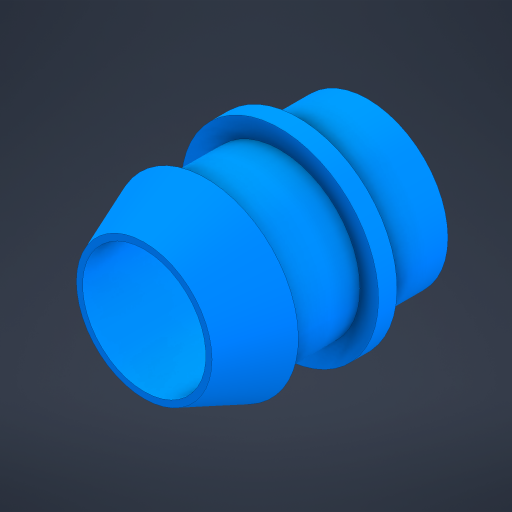
# Autodesk Inventor part: servo_rod_outlet
Saved by Autodesk Inventor 2023 (Build 270158030, 158C)
## iProperties
Created: 2023-02-26
Part Number: servo_rod_outlet
Material: Generic
Document SubType Name: Modeling
Designer: kardo
Density: 1 g/cm^3
Appearance: Blue Plastic
Author: kardo
Autodesk Inventor part; units mm, degrees
ref_plane "YZ Plane" through (0, 0, 0) normal (1, 0, 0) x (0, 1, 0)
ref_plane "XZ Plane" through (0, 0, 0) normal (0, 1, 0) x (-1, 0, 0)
ref_plane "XY Plane" through (0, 0, 0) normal (0, 0, 1) x (1, 0, 0)
derived "parameters_frame.ipt"
sketch "sk_profile" plane through (0, 0, 0) normal (1, 0, 0) x (0, 1, 0)
  line L0 (0, -7.4) -> (0, 12.9) construction
  line L1 (-7.68, 0) -> (1.28, 0) construction
  line L2 (-4, 10) -> (-4, -4.5)
  line L3 (-4, -4.5) -> (-5.2, -4.5)
  line L4 (-5.2, -4.5) -> (-5.2, 0)
  line L5 (-5.2, 0) -> (-6.4, 0)
  line L6 (-6.4, 0) -> (-6.4, 1.2)
  line L7 (-6.4, 1.2) -> (-5.2, 1.2)
  line L8 (-5.2, 1.2) -> (-5.2, 6)
  line L9 (-5.2, 6) -> (-6, 6)
  line L10 (-6, 6) -> (-4.4, 10)
  line L11 (-4.4, 10) -> (-4, 10)
  point P0 (0, 0)
  dimension "d8" = 1.2
  dimension "d9" = 5.2
  dimension "d10" = 1.2
  dimension "d11" = 1.2
  dimension "d12" = 4.8
  dimension "d13" = 4
  dimension "d14" = 0.4
  dimension "d15" = 0.8
  dimension "d16" = 4.5
  constraints: 20 end point, 5 perpendicular, 4 parallel, 2 collinear
  measures "d8" distance of L2.end L3.end
  measures "d9" distance between parallel lines of L0 L4
  measures "d10" distance of L5.end L6.end
  measures "d11" distance between parallel lines of L4 L6
  measures "d12" distance of L7.end L8.end
  measures "d13" distance between parallel lines of L11 L9
  measures "d14" distance of L10.end L2.start
  measures "d15" distance of L8.end L9.end
  measures "d16" distance between parallel lines of L1 L3
revolve "body" add sketch "sk_profile" angle 360 about axis through (0, 0, -10) along (0, 0, 1)
equation "\"d9\" = 0.5 * drill_servo_rod_diam"
equation "\"drill_servo_rod_diam\" = 10.4"
body "Solid2"
